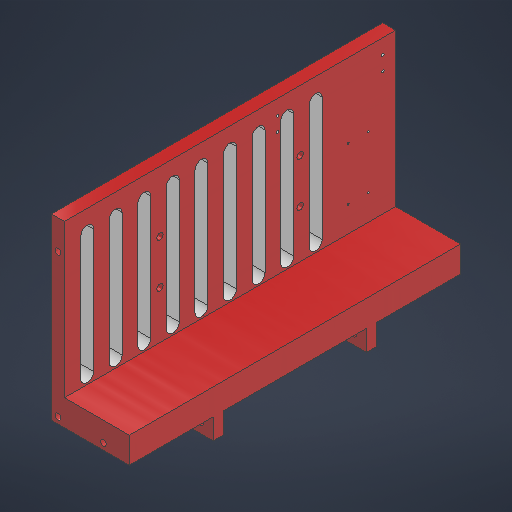
# Autodesk Inventor part: EboxCase
Saved by Autodesk Inventor 2025.1 (Build 291241000, 241)
## iProperties
Created: 2025-02-21
Part Number: EboxCase
Material: Generic
Document SubType Name: Modeling
Designer: m_kni
Density: 1 g/cm^3
Appearance: Default
Finish1_Area: 90514.407 mm^2
Finish1_Appearance: Red
Finish1_Process: Prime/Paint RAL 3018
Finish1_Description: Prime/Paint RAL 3018
Finish1_ShortDescription: RAL 3018
Finish1_Thickness: 0.050 mm
Author: m_kni
## iProperties of the stored document EboxCase_3DPrint.ipt
Created: 2025-03-29
Part Number: EboxCase_3DPrint
Material: Generic
Document SubType Name: Modeling
Designer: m_kni
Density: 1 g/cm^3
Appearance: Default
Author: m_kni
Autodesk Inventor part; units mm, degrees
ref_plane "YZ Plane" through (0, 0, 0) normal (1, 0, 0) x (0, 1, 0)
ref_plane "XZ Plane" through (0, 0, 0) normal (0, 1, 0) x (-1, 0, 0)
sketch "Sketch1" plane through (0, 0, 0) normal (0, 1, 0) x (-1, 0, 0)
  line L0 (-75, -127.5) -> (75, -127.5)
  line L1 (75, -127.5) -> (75, 127.5)
  line L2 (75, 127.5) -> (-75, 127.5)
  line L3 (-75, 127.5) -> (-75, -127.5)
  line L4 (-75, -127.5) -> (75, 127.5) construction
  line L5 (75, -127.5) -> (-75, 127.5) construction
  line L6 (-75, 0) -> (-36.5, 0)
  line L7 (-41.5, -127.5) -> (-31.5, -127.5)
  line L8 (-31.5, -127.5) -> (-31.5, 127.5)
  line L9 (-31.5, 127.5) -> (-41.5, 127.5)
  line L10 (-41.5, 127.5) -> (-41.5, -127.5)
  line L11 (-41.5, -127.5) -> (-31.5, 127.5) construction
  line L12 (-31.5, -127.5) -> (-41.5, 127.5) construction
  line L13 (12.5, -127.5) -> (22.5, -127.5)
  line L14 (22.5, -127.5) -> (22.5, 127.5)
  line L15 (22.5, 127.5) -> (12.5, 127.5)
  line L16 (12.5, 127.5) -> (12.5, -127.5)
  line L17 (12.5, -127.5) -> (22.5, 127.5) construction
  line L18 (22.5, -127.5) -> (12.5, 127.5) construction
  line L19 (75, 127.5) -> (22.1863, 127.5)
  line L20 (22.1863, 127.5) -> (22.1863, 119.5)
  line L21 (22.1863, 119.5) -> (75, 119.5)
  line L22 (75, 119.5) -> (75, 127.5)
  line L23 (75, -127.5) -> (22.1863, -127.5)
  line L24 (22.1863, -127.5) -> (22.1863, -119.5)
  line L25 (22.1863, -119.5) -> (75, -119.5)
  line L26 (75, -119.5) -> (75, -127.5)
  line L27 (12.8137, -119.5) -> (-31.5, -119.5)
  line L28 (-31.5, -119.5) -> (-31.5, -127.5)
  line L29 (-31.5, -127.5) -> (12.8137, -127.5)
  line L30 (12.8137, -127.5) -> (12.8137, -119.5)
  line L31 (22.1863, 119.5) -> (-31.5, 119.5)
  line L32 (-31.5, 119.5) -> (-31.5, 127.5)
  line L33 (-31.5, 127.5) -> (22.1863, 127.5)
  line L34 (22.1863, 127.5) -> (22.1863, 119.5)
  point P0 (0, 0)
  point P1 (17.5, 0)
  point P2 (22.5, -119.5)
  point P3 (22.5, 119.5)
  point P4 (-31.5, -119.5)
  point P5 (12.5, 119.5)
  point P6 (12.5, -119.5)
  dimension "d0" = 150
  dimension "d1" = 255
  dimension "d3" = 10
  dimension "d4" = 92.5
  dimension "d5" = 10
  dimension "d6" = 8
  dimension "d7" = 8
  constraints: 70 end point, 14 parallel, 8 horizontal, 7 midpoint, 7 perpendicular, 5 point on line
  measures "d0" distance of L2.end L1.end
  measures "d1" distance of L1.end L0.end
  measures "d3" distance of L9.end L8.end
  measures "d4" distance from line of point (17.5, 0) L3
  measures "d5" distance of L15.end L14.end
  measures "d6" distance of L20.end L19.end
  measures "d7" distance of L23.end L24.end
extrude "Extrusion1" add sketch "Sketch1" along normal blind 5
extrude "Extrusion2" add sketch "Sketch1" against normal blind 147.5 contours L10 L2 L8 L0 | L8 L27 L16 L0 | L16 L27 L30 L0 | L30 L27 L16 L31 L21 L14 L25 L24 L0 | L8 L2 L16 L31 | L24 L25 L14 L0 | L16 L2 L20 L31 | L14 L25 L1 L0 | L20 L2 L14 L21 | L14 L2 L1 L21
sketch "Sketch2" plane through (41.5, -147.5, 127.5) normal (1, 0, 0) x (0, 0, -1)
  line L0 (255, 152.5) -> (255, 0) projected
  line L1 (0, 0) -> (0, 152.5) projected
  line L2 (255, 0) -> (0, 0)
  line L3 (0, 0) -> (0, 147.5)
  line L4 (0, 147.5) -> (255, 147.5)
  line L5 (255, 147.5) -> (255, 0)
  line L6 (255, 73.75) -> (0, 73.75)
  line L7 (127.5, 73.75) -> (127.5, 36.343)
  line L8 (73.5, 73.75) -> (73.5, 56.75)
  line L9 (181.5, 73.75) -> (181.5, 56.75)
  line L10 (73.5, 73.75) -> (73.5, 90.75)
  line L11 (181.5, 73.75) -> (181.5, 90.75)
  circle A0 centre (181.5, 56.75) radius 2.5
  circle A1 centre (181.5, 90.75) radius 2.5
  circle A2 centre (73.5, 90.75) radius 2.5
  circle A3 centre (73.5, 56.75) radius 2.5
  point P0 (127.5, 147.5)
  point P1 (127.5, 55.0465)
  point P2 (73.5, 60.2872)
  dimension "d12" = 54
  dimension "d13" = 17
  dimension "d14" = 5
  dimension "d15" = 5
  dimension "d16" = 5
  dimension "d17" = 5
  constraints: 20 end point, 4 centre point, 4 coincident, 4 midpoint, 4 symmetric about line, 2 parallel, 2 point on line, 2 vertical, 1 horizontal, 1 perpendicular
  measures "d12" horizontal distance of L8.start point (127.5, 55.047)
  measures "d13" distance of L8.start L8.end
  measures "d14" diameter of A0
  measures "d15" diameter of A1
  measures "d16" diameter of A2
  measures "d17" diameter of A3
extrude "Extrusion3" cut sketch "Sketch2" against normal blind 147.5 contours A0 | A1 | A2 | A3
sketch "Sketch3" plane through (-22.5, -147.5, -119.5) normal (-1, 0, 0) x (0, 0, 1)
  point P0 (119.5, 147.5)
sketch "Sketch4" plane through (-22.5, -147.5, -119.5) normal (-1, 0, 0) x (0, 0, 1)
  circle A0 centre (173.5, 90.75) radius 2.5 projected
  circle A1 centre (173.5, 56.75) radius 2.5 projected
  circle A2 centre (65.5, 90.75) radius 2.5 projected
  circle A3 centre (65.5, 56.75) radius 2.5 projected
  circle A4 centre (173.5, 90.75) radius 5
  circle A5 centre (173.5, 56.75) radius 5
  circle A6 centre (65.5, 90.75) radius 5
  circle A7 centre (65.5, 56.75) radius 5
  line L0 (237, 10) -> (77, 10)
  line L1 (77, 10) -> (77, 110)
  line L2 (77, 110) -> (237, 110)
  line L3 (237, 110) -> (237, 10)
  line L4 (237, 10) -> (77, 110) construction
  line L5 (77, 10) -> (237, 110) construction
  line L6 (239, 147.5) -> (239, 0) projected
  line L7 (239, 0) -> (0, 0) projected
  line L8 (3, 106.5) -> (67, 106.5)
  line L9 (67, 106.5) -> (67, 13.5)
  line L10 (67, 13.5) -> (3, 13.5)
  line L11 (3, 13.5) -> (3, 106.5)
  line L12 (3, 106.5) -> (67, 13.5) construction
  line L13 (67, 106.5) -> (3, 13.5) construction
  line L14 (157, 60) -> (147.6244, 60)
  line L15 (147.6244, 60) -> (147.6244, 51.0165)
  line L16 (157, 60) -> (157, 51.0165)
  circle A8 centre (232, 15.5) radius 1.5
  circle A9 centre (232, 104.5) radius 1.5
  circle A10 centre (82, 15.5) radius 1.5
  circle A11 centre (82, 104.5) radius 1.5
  point P0 (119.5, 147.5)
  point P1 (35, 60)
  point P2 (157, 10)
  point P3 (232, 10)
  point P4 (82, 10)
  dimension "d20" = 10
  dimension "d21" = 10
  dimension "d22" = 10
  dimension "d23" = 10
  dimension "d24" = 160
  dimension "d25" = 100
  dimension "d26" = 82
  dimension "d27" = 60
  dimension "d28" = 64
  dimension "d29" = 93
  dimension "d30" = 10
  dimension "d31" = 75
  dimension "d32" = 75
  dimension "d33" = 44.5
  dimension "d34" = 3
  dimension "d35" = 3
  dimension "d36" = 3
  dimension "d37" = 3
  constraints: 30 end point, 8 centre point, 8 coincident, 5 midpoint, 4 parallel, 3 horizontal, 3 perpendicular, 3 symmetric about line, 2 point on line, 1 vertical
  measures "d20" diameter of A4
  measures "d21" diameter of A5
  measures "d22" diameter of A6
  measures "d23" diameter of A7
  measures "d24" distance of L1.end L2.end
  measures "d25" distance of L0.end L1.end
  measures "d26" distance from line of L14.start L6
  measures "d27" distance from line of L14.start L7
  measures "d28" distance of L9.end L10.end
  measures "d29" distance of L8.end L9.end
  measures "d30" distance between parallel lines of L9 L1
  measures "d31" distance of point (232, 10) point (157, 10)
  measures "d32" distance of point (82, 10) point (157, 10)
  measures "d33" vertical distance of point (232, 15.5) L14.start
  measures "d34" diameter of A8
  measures "d35" diameter of A9
  measures "d36" diameter of A10
  measures "d37" diameter of A11
extrude "Extrusion4" cut sketch "Sketch4" against normal blind 10 contours A8 | A9 | A10 | A11
sketch "Sketch5" plane through (-75, 5, 127.5) normal (0, 0, 1) x (1, 0, 0)
  line L0 (150, -5) -> (118.233, -36.767)
  line L1 (150, -5) -> (194.9254, -5) construction
  line L2 (118.233, -36.767) -> (116.5, -38.5)
  line L3 (116.5, -5) -> (116.5, -152.5) projected
  line L4 (116.5, -152.5) -> (116.5, -132.5)
  line L5 (116.5, -132.5) -> (166.5, -132.5)
  line L6 (116.5, -152.5) -> (166.5, -152.5)
  line L7 (166.5, -152.5) -> (166.5, -132.5)
  line L8 (116.5, -5) -> (150, -5) projected
  line L9 (150, -5) -> (150, 0) projected
  line L10 (0, 0) -> (150, 0) projected
  line L11 (0, -152.5) -> (0, 0) projected
  line L12 (116.5, -152.5) -> (0, -152.5) projected
  line L13 (116.5, -5) -> (116.5, -152.5) projected
  line L14 (166.5, -132.5) -> (116.5, -82.5)
  point P0 (75, -5)
  dimension "d40" = 135
  dimension "d41" = 20
  dimension "d42" = 50
  constraints: 16 end point, 4 point on line, 3 horizontal, 1 equal length, 1 perpendicular
  measures "d40" angle of L0 L1
  measures "d41" distance of L3.end L4.end
  measures "d42" distance of L4.end L5.end
extrude "Extrusion5" add sketch "Sketch5" along normal blind 10
ref_plane "Work Plane1" through (-22.5, 0, 0) normal (0, 0, -1) x (-1, 0, 0)
mirror "Mirror1" about plane through (-22.5, 0, 0) normal (0, 0, -1) of "Extrusion5"
extrude "Extrusion6" add sketch "Sketch5" against normal up to surface (255 mm away) contours L5 L7 L6 L3
sketch "Sketch6" plane through (0, 0, 0) normal (0, -1, 0) x (1, 0, 0)
  line L0 (75, 127.5) -> (75, -127.5) projected
  line L1 (41.5, 127.5) -> (75, 127.5) projected
  circle A0 centre (61.5, -85.5) radius 1.5
  circle A1 centre (61.5, 64.5) radius 1.5
  point P0 (0, 0)
  dimension "d47" = 13.5
  dimension "d48" = 63
  dimension "d49" = 150
  dimension "d50" = 3
  dimension "d51" = 3
  constraints: 2 centre point, 2 coincident
  measures "d47" distance from line of point (61.5, 64.5) L0
  measures "d48" distance from line of point (61.5, 64.5) L1
  measures "d49" distance of point (61.5, -85.5) point (61.5, 64.5)
  measures "d50" diameter of A0
  measures "d51" diameter of A1
extrude "Extrusion7" cut sketch "Sketch6" against normal blind 10
sketch "Sketch7" plane through (0, 5, 0) normal (0, 1, 0) x (1, 0, 0)
  circle A0 centre (61.5, -64.5) radius 1.5 projected
  circle A1 centre (61.5, 85.5) radius 1.5 projected
  line L0 (-75, -137.5) -> (-75, 137.5) projected
  line L1 (75, -137.5) -> (-75, -137.5) projected
  line L2 (75, 137.5) -> (75, -137.5) projected
  line L3 (75, 137.5) -> (-75, 137.5) projected
  point P0 (0, 0)
extrude "Extrusion8" cut sketch "Sketch7" against normal up to surface (5 mm away)
sketch "Sketch8" plane through (41.5, 0, 127.5) normal (0, 1, 0) x (1, 0, 0)
  line L0 (-10, 8) -> (-54, 8) projected
  line L1 (-54, 8) -> (-54, 247) projected
  line L2 (-54, 247) -> (-10, 247) projected
  line L3 (-10, 247) -> (-10, 8) projected
  line L4 (-64, 8) -> (-116.5, 8) projected
  line L5 (-116.5, -10) -> (-116.5, 8) projected
  line L6 (33.5, -10) -> (-116.5, -10) projected
  line L7 (33.5, 0) -> (33.5, -10) projected
  line L8 (0, 0) -> (33.5, 0) projected
  line L9 (0, 0) -> (0, 255) projected
  line L10 (33.5, 255) -> (0, 255) projected
  line L11 (33.5, 255) -> (33.5, 265) projected
  line L12 (-116.5, 265) -> (33.5, 265) projected
  line L13 (-116.5, 247) -> (-116.5, 265) projected
  line L14 (-116.5, 247) -> (-64, 247) projected
  line L15 (-64, 247) -> (-64, 8) projected
  circle A0 centre (-96.5, 260) radius 1
  circle A1 centre (13.5, 260) radius 1
  circle A2 centre (-96.5, -5) radius 1
  circle A3 centre (13.5, -5) radius 1
  point P0 (-41.5, 127.5)
  point P1 (33.5, 260)
  point P2 (33.5, -5)
  dimension "d56" = 20
  dimension "d57" = 20
  dimension "d58" = 20
  dimension "d59" = 20
  dimension "d60" = 2
  dimension "d61" = 2
  dimension "d62" = 2
  dimension "d63" = 2
  constraints: 4 centre point, 4 coincident, 2 midpoint
  measures "d56" distance from line of point (-96.5, 260) L13
  measures "d57" distance of point (13.5, 260) point (33.5, 260)
  measures "d58" distance from line of point (-96.5, -5) L5
  measures "d59" distance of point (13.5, -5) point (33.5, -5)
  measures "d60" diameter of A0
  measures "d61" diameter of A1
  measures "d62" diameter of A2
  measures "d63" diameter of A3
extrude "Extrusion9" cut sketch "Sketch8" against normal blind 10 contours A0 | A1 | A2 | A3
sketch "Sketch9" plane through (0, -147.5, 0) normal (0, -1, 0) x (1, 0, 0)
  line L0 (91.5, 127.5) -> (91.5, -127.5) projected
  line L1 (91.5, 0) -> (91.5, -55)
  line L2 (91.5, 0) -> (91.5, 55)
  line L3 (91.5, 55) -> (71.5, 55)
  line L4 (91.5, -55) -> (71.5, -55)
  line L5 (71.5, 55) -> (91.5, 55)
  line L6 (91.5, 55) -> (91.5, 63)
  line L7 (91.5, 63) -> (71.5, 63)
  line L8 (71.5, 63) -> (71.5, 55)
  line L9 (91.5, -55) -> (71.5, -55)
  line L10 (71.5, -55) -> (71.5, -63)
  line L11 (71.5, -63) -> (91.5, -63)
  line L12 (91.5, -63) -> (91.5, -55)
  point P0 (0, 0)
  dimension "d66" = 55
  dimension "d67" = 55
  dimension "d68" = 20
  dimension "d69" = 20
  dimension "d70" = 8
  dimension "d71" = 8
  constraints: 24 end point, 4 parallel, 3 horizontal, 3 perpendicular, 3 point on line, 1 midpoint
  measures "d66" distance of L1.start L1.end
  measures "d67" distance of L1.start L2.end
  measures "d68" distance of L2.end L3.end
  measures "d69" distance of L1.end L4.end
  measures "d70" distance of L3.end L7.end
  measures "d71" distance of L10.end L9.end
extrude "Extrusion10" add sketch "Sketch9" along normal blind 16
sketch "Sketch10" plane through (71.5, -147.5, 63) normal (0, 0, 1) x (1, 0, 0)
  line L0 (0, 0) -> (20, 0) projected
  line L1 (0, 0) -> (0, -16) projected
  line L2 (20, -16) -> (0, -16) projected
  line L3 (20, 0) -> (20, -16) projected
  line L4 (20, -16) -> (0, -16)
  line L5 (0, -16) -> (0, 0)
  line L6 (0, 0) -> (20, 0)
  line L7 (20, 0) -> (20, -16)
  circle A0 centre (10, -8) radius 2.6
  point P0 (-71.5, 147.5)
  dimension "d74" = 5.2
  constraints: 8 end point, 2 parallel, 1 centre point, 1 horizontal, 1 perpendicular
  measures "d74" diameter of A0
extrude "Extrusion11" cut sketch "Sketch10" against normal blind 144.5875 contours A0
fillet "Fillet1" radius 62.325 2 edges at (71.5, -147.5, 59) (71.5, -147.5, -59)
sketch "Sketch11" plane through (-75, 5, 137.5) normal (0, 0, 1) x (1, 0, 0)
  line L0 (0, -5) -> (0, -152.5) projected
  line L1 (0, -5) -> (0, -152.5)
  line L2 (150, -5) -> (0, -5) projected
  line L3 (0, -5) -> (0, -152.5) projected
  line L4 (0, -152.5) -> (166.5, -152.5) projected
  line L5 (166.5, -152.5) -> (166.5, -132.5) projected
  line L6 (166.5, -132.5) -> (116.5, -82.5) projected
  line L7 (116.5, -82.5) -> (116.5, -38.5) projected
  line L8 (116.5, -38.5) -> (150, -5) projected
  point P0 (75, -5)
  constraints: 2 end point, 1 vertical
extrude "Extrusion12" cut sketch "Sketch11" against normal blind 10
mirror "Mirror2" about plane through (-22.5, 0, 0) normal (0, 0, -1) of "Extrusion12"
sketch "Sketch13" plane through (-75, 5, 127.5) normal (0, 0, 1) x (1, 0, 0)
  line L0 (0, -5) -> (0, -152.5) projected
  line L1 (52.5, -5) -> (52.5, -152.5) projected
  line L2 (0, -152.5) -> (52.5, -152.5)
  line L3 (52.5, -152.5) -> (52.5, -5)
  line L4 (52.5, -5) -> (0, -5)
  line L5 (0, -5) -> (0, -152.5)
  point P0 (75, -5)
  constraints: 8 end point, 2 parallel, 1 horizontal, 1 perpendicular
extrude "Extrusion13" cut sketch "Sketch13" against normal blind 437.675
sketch "Sketch14" plane through (0, -147.5, 0) normal (0, -1, 0) x (1, 0, 0)
  line L0 (31.5, -119.5) -> (-12.5, -119.5) projected
  line L1 (-22.5, -127.5) -> (91.5, -127.5) projected
  line L2 (31.5, -119.5) -> (-12.5, -119.5)
  line L3 (-12.5, -119.5) -> (-12.5, -127.5)
  line L4 (-12.5, -127.5) -> (31.5, -127.5)
  line L5 (31.5, -127.5) -> (31.5, -119.5)
  line L6 (-22.5, 127.5) -> (41.5, 127.5) projected
  line L7 (31.5, -127.5) -> (-12.5, -127.5)
  line L8 (-12.5, -127.5) -> (-12.5, 127.5)
  line L9 (-12.5, 127.5) -> (31.5, 127.5)
  line L10 (31.5, 127.5) -> (31.5, -127.5)
  point P0 (0, 0)
  dimension "d82" = 44
  constraints: 16 end point, 4 parallel, 2 horizontal, 2 perpendicular, 2 point on line
  measures "d82" distance of L4.end L3.end
extrude "Extrusion14" cut sketch "Sketch14" against normal blind 437.675
sketch "Sketch15" plane through (-22.5, -147.5, 127.5) normal (-1, 0, 0) x (0, 0, 1)
  circle A0 centre (-165, 15.5) radius 1.5 projected
  circle A1 centre (-15, 104.5) radius 1.5 projected
  circle A2 centre (-165, 104.5) radius 1.5 projected
  circle A3 centre (-15, 15.5) radius 1.5 projected
  circle A4 centre (-73.5, 56.75) radius 2.5 projected
  circle A5 centre (-181.5, 90.75) radius 2.5 projected
  circle A6 centre (-73.5, 90.75) radius 2.5 projected
  circle A7 centre (-181.5, 56.75) radius 2.5 projected
  line L0 (-255, 147.5) -> (0, 147.5) projected
  line L1 (-255, 0) -> (-255, 147.5) projected
  line L2 (0, 0) -> (-255, 0) projected
  line L3 (0, 147.5) -> (0, 0) projected
  point P0 (-127.5, 147.5)
extrude "Extrusion15" cut sketch "Sketch15" against normal blind 10
sketch "Sketch16" plane through (-75, 5, 127.5) normal (0, 0, 1) x (1, 0, 0)
  line L0 (166.5, -132.5) -> (166.5, -152.5) projected
  line L1 (166.5, -152.5) -> (106.5, -152.5) projected
  circle A0 centre (146.5, -147.5) radius 2.25
  circle A1 centre (111.5, -147.5) radius 2.25
  circle A2 centre (111.5, -10) radius 2.25
  line L2 (106.5, -5) -> (116.5, -5) projected
  circle A3 centre (111.5, -37.5) radius 2.25
  point P0 (75, -5)
  dimension "d87" = 20
  dimension "d88" = 5
  dimension "d89" = 4.5
  dimension "d92" = 4.5
  dimension "d93" = 35
  dimension "d94" = 4.5
  dimension "d95" = 5
  dimension "d97" = 4.5
  dimension "d98" = 110
  constraints: 4 centre point, 1 coincident
  measures "d87" distance from line of point (146.5, -147.5) L0
  measures "d88" distance from line of L1 point (146.5, -147.5)
  measures "d89" diameter of A0
  measures "d92" diameter of A1
  measures "d93" distance of A1.centre A0.centre
  measures "d94" diameter of A2
  measures "d95" distance from line of L2 A2.centre
  measures "d97" diameter of A3
  measures "d98" distance of A1.centre A3.centre
extrude "Extrusion16" cut sketch "Sketch16" against normal blind 6 contours A0 | A1 | A3
mirror "Mirror3" about plane through (-22.5, 0, 0) normal (0, 0, -1) of "Extrusion16"
extrude "Extrusion17" cut sketch "Sketch1" against normal blind 10 contours L10 L2 L8 L0
sketch "Sketch17" plane through (41.5, -127.5, 127.5) normal (1, 0, 0) x (0, 0, -1)
  line L0 (255, 117.5) -> (0, 117.5) projected
  line L1 (255, 117.5) -> (0, 117.5) projected
  line L2 (0, 117.5) -> (0, 0) projected
  line L3 (0, 0) -> (255, 0) projected
  line L4 (255, 117.5) -> (255, 0) projected
  circle A0 centre (73.5, 36.75) radius 2.5 projected
  circle A1 centre (181.5, 70.75) radius 2.5 projected
  circle A2 centre (73.5, 70.75) radius 2.5 projected
  circle A3 centre (181.5, 36.75) radius 2.5 projected
  line L5 (255, 117.5) -> (0, 117.5)
  line L6 (0, 117.5) -> (0, 0)
  line L7 (0, 0) -> (255, 0)
  line L8 (255, 0) -> (255, 117.5)
  line L9 (250, -1.25) -> (5, -1.25)
  line L10 (5, -1.25) -> (5, 108.75)
  line L11 (5, 108.75) -> (250, 108.75)
  line L12 (250, 108.75) -> (250, -1.25)
  line L13 (250, -1.25) -> (5, 108.75) construction
  line L14 (5, -1.25) -> (250, 108.75) construction
  point P0 (127.5, 127.5)
  point P1 (127.5, 117.5)
  point P2 (255, 58.75)
  point P3 (127.5, 53.75)
  dimension "d101" = 245
  dimension "d102" = 110
  constraints: 20 end point, 4 midpoint, 4 parallel, 2 horizontal, 2 perpendicular
  measures "d101" distance of L10.end L11.end
  measures "d102" distance of L9.end L10.end
sketch "Sketch18" plane through (31.5, -147.5, -55) normal (-1, 0, 0) x (0, 0, 1)
  line L0 (-51.4025, 80.3931) -> (-35.9825, 80.3931)
  line L1 (-35.9825, 80.3931) -> (-35.9825, 39.7531)
  line L2 (-35.9825, 39.7531) -> (-51.4025, 39.7531)
  line L3 (-51.4025, 39.7531) -> (-51.4025, 80.3931)
  line L4 (-51.4025, 80.3931) -> (-35.9825, 39.7531) construction
  line L5 (-35.9825, 80.3931) -> (-51.4025, 39.7531) construction
  circle A0 centre (-35.9825, 39.7531) radius 0.75
  circle A1 centre (-51.4025, 39.7531) radius 0.75
  circle A2 centre (-35.9825, 80.3931) radius 0.75
  circle A3 centre (-51.4025, 80.3931) radius 0.75
  point P0 (55, 147.5)
  point P1 (-43.6925, 60.0731)
  dimension "d103" = 15.42
  dimension "d104" = 40.64
  dimension "d105" = 1.5
  dimension "d106" = 1.5
  dimension "d107" = 1.5
  dimension "d108" = 1.5
  constraints: 12 end point, 4 centre point, 4 coincident, 2 midpoint, 2 parallel, 1 horizontal, 1 perpendicular
  measures "d103" distance of L1.end L2.end
  measures "d104" distance of L0.end L1.end
  measures "d105" diameter of A0
  measures "d106" diameter of A1
  measures "d107" diameter of A2
  measures "d108" diameter of A3
extrude "Extrusion18" cut sketch "Sketch18" against normal blind 10 contours L3 A3 L0 | L0 A3 L3 | A2 L1 L0 | L0 L1 A2 | A1 L2 L3 | L3 L2 A1 | A0 L2 L1 | L1 L2 A0
sketch "Sketch19" plane through (31.5, -147.5, -55) normal (-1, 0, 0) x (0, 0, 1)
  line L0 (-62.6322, 115.0616) -> (18.3678, 115.0616)
  line L1 (18.3678, 115.0616) -> (18.3678, 126.0616)
  line L2 (18.3678, 126.0616) -> (-62.6322, 126.0616)
  line L3 (-62.6322, 126.0616) -> (-62.6322, 115.0616)
  circle A0 centre (-62.6322, 115.0616) radius 1
  circle A1 centre (-62.6322, 126.0616) radius 1
  circle A2 centre (18.3678, 126.0616) radius 1
  circle A3 centre (18.3678, 115.0616) radius 1
  point P0 (55, 147.5)
  dimension "d111" = 81
  dimension "d112" = 11
  dimension "d113" = 2
  dimension "d114" = 2
  dimension "d115" = 2
  dimension "d116" = 2
  constraints: 8 end point, 4 centre point, 4 coincident, 2 parallel, 1 horizontal, 1 perpendicular
  measures "d111" distance of L2.end L1.end
  measures "d112" distance of L1.end L0.end
  measures "d113" diameter of A0
  measures "d114" diameter of A1
  measures "d115" diameter of A2
  measures "d116" diameter of A3
extrude "Extrusion19" cut sketch "Sketch19" against normal blind 10 contours L3 A0 L0 | L0 A0 L3 | A3 L1 L0 | L0 L1 A3 | A1 L2 L3 | L3 L2 A1 | A2 L2 L1 | L1 L2 A2
sketch "Sketch20" plane through (41.5, -127.5, 127.5) normal (1, 0, 0) x (0, 0, -1)
  line L0 (5, -1.25) -> (250, 108.75) construction
  line L1 (250, -1.25) -> (5, 108.75) construction
  line L2 (237.5, 6.25) -> (17.5, 6.25)
  line L3 (17.5, 6.25) -> (17.5, 101.25)
  line L4 (17.5, 101.25) -> (237.5, 101.25)
  line L5 (237.5, 101.25) -> (237.5, 6.25)
  line L6 (237.5, 6.25) -> (17.5, 101.25) construction
  line L7 (17.5, 6.25) -> (237.5, 101.25) construction
  circle A0 centre (17.5, 101.25) radius 5
  circle A1 centre (17.5, 6.25) radius 5
  line L8 (22.5, 101.25) -> (22.5, 6.25)
  line L9 (12.5, 6.25) -> (12.5, 101.25)
  line L10 (44.5, 101.25) -> (44.5, 6.25)
  circle A2 centre (39.5, 101.25) radius 5
  circle A3 centre (39.5, 6.25) radius 5
  line L11 (34.5, 6.25) -> (34.5, 101.25)
  line L12 (66.5, 101.25) -> (66.5, 6.25)
  circle A4 centre (61.5, 101.25) radius 5
  circle A5 centre (61.5, 6.25) radius 5
  line L13 (56.5, 6.25) -> (56.5, 101.25)
  line L14 (88.5, 101.25) -> (88.5, 6.25)
  circle A6 centre (83.5, 101.25) radius 5
  circle A7 centre (83.5, 6.25) radius 5
  line L15 (78.5, 6.25) -> (78.5, 101.25)
  line L16 (110.5, 101.25) -> (110.5, 6.25)
  circle A8 centre (105.5, 101.25) radius 5
  circle A9 centre (105.5, 6.25) radius 5
  line L17 (100.5, 6.25) -> (100.5, 101.25)
  line L18 (132.5, 101.25) -> (132.5, 6.25)
  circle A10 centre (127.5, 101.25) radius 5
  circle A11 centre (127.5, 6.25) radius 5
  line L19 (122.5, 6.25) -> (122.5, 101.25)
  line L20 (154.5, 101.25) -> (154.5, 6.25)
  circle A12 centre (149.5, 101.25) radius 5
  circle A13 centre (149.5, 6.25) radius 5
  line L21 (144.5, 6.25) -> (144.5, 101.25)
  line L22 (176.5, 101.25) -> (176.5, 6.25)
  circle A14 centre (171.5, 101.25) radius 5
  circle A15 centre (171.5, 6.25) radius 5
  line L23 (166.5, 6.25) -> (166.5, 101.25)
  line L24 (198.5, 101.25) -> (198.5, 6.25)
  circle A16 centre (193.5, 101.25) radius 5
  circle A17 centre (193.5, 6.25) radius 5
  line L25 (188.5, 6.25) -> (188.5, 101.25)
  point P0 (127.5, 127.5)
  point P1 (127.5, 53.75)
  dimension "d119" = 220
  dimension "d120" = 95
  dimension "d121" = 10
  dimension "d122" = 10
  dimension "d125" = 22
  constraints: 48 end point, 36 point on circle, 18 centre point, 3 midpoint, 3 parallel, 2 coincident, 2 horizontal, 2 point on line, 1 perpendicular, 1 tangent, 80 other
  measures "d119" distance of L3.end L4.end
  measures "d120" distance of L2.end L3.end
  measures "d121" diameter of A0
  measures "d122" diameter of A1
  measures "d125" distance of L8.start L10.start
extrude "Extrusion20" cut sketch "Sketch20" against normal blind 10 contours A17 L2 | A17 L25 A16 L24 | L2 A17 | A16 L4 | L4 A16 | A15 L2 | A15 L23 A14 L22 | L2 A15 | A14 L4 | L4 A14 | A13 L2 | A13 L21 A12 L20 | L2 A13 | A12 L4 | L4 A12 | A11 L2 | A11 L19 A10 L18 | L2 A11 | A10 L4 | L4 A10 | A9 L2 | A9 L17 A8 L16 | L2 A9 | A8 L4 | L4 A8 | A7 L2 | A7 L15 A6 L14 | L2 A7 | A6 L4 | L4 A6 | A5 L2 | A5 L13 A4 L12 | L2 A5 | A4 L4 | L4 A4 | A3 L2 | A3 L11 A2 L10 | L2 A3 | A2 L4 | L4 A2 | A1 L3 L2 | L2 L3 A1 | A1 L3 A0 L8 | L9 A0 L3 A1 | A0 L3 L4 | L4 L3 A0
ref_plane "Work Plane2" through (-22.5, 0, 0) normal (0, 0, -1) x (-1, 0, 0)
body "Solid1"
